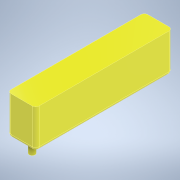
# Autodesk Inventor part: Schmierung
Saved by Autodesk Inventor 2022 (Build 260153000, 153)
## iProperties
Created: 2023-01-30
Part Number: Schmierung
Material: Wasser
Document SubType Name: Modeling
Designer: Matias Nicky
Density: 0.9983 g/cm^3
Appearance: Gelb
Author: Matias Nicky
Autodesk Inventor part; units mm, degrees
ref_plane "YZ Plane" through (0, 0, 0) normal (1, 0, 0) x (0, 1, 0)
ref_plane "XZ Plane" through (0, 0, 0) normal (0, 1, 0) x (-1, 0, 0)
ref_plane "XY Plane" through (0, 0, 0) normal (0, 0, 1) x (1, 0, 0)
sketch "Skizze1" plane through (0, 0, 0) normal (0, 1, 0) x (-1, 0, 0)
  line L0 (-15, -97) -> (15, -97)
  line L1 (20, -92) -> (20, 92)
  line L2 (15, 97) -> (-15, 97)
  line L3 (-20, 92) -> (-20, -92)
  line L4 (-20, -97) -> (20, 97) construction
  line L5 (20, -97) -> (-20, 97) construction
  arc A0 (20, 95) -> (18, 97) centre (18, 95) ccw
  arc A1 (20, 92) -> (15, 97) centre (15, 92) ccw
  arc A2 (-15, 97) -> (-20, 92) centre (-15, 92) ccw
  arc A3 (-20, -92) -> (-15, -97) centre (-15, -92) ccw
  arc A4 (15, -97) -> (20, -92) centre (15, -92) ccw
  point P0 (0, 0)
  dimension "d0" = 40
  dimension "d1" = 194
  dimension "d3" = 5
  dimension "d4" = 5
  constraints: 12 end point, 10 point on circle, 10 point on line, 10 tangent, 5 centre point, 2 equal radius, 2 midpoint, 2 parallel, 1 horizontal, 1 perpendicular
  measures "d0" distance of L5.end L4.end
  measures "d1" distance of L5.start L4.end
  measures "d3" radius of A1
  measures "d4" radius of A2
extrude "Extrusion1" add sketch "Skizze1" along normal blind 55
sketch "Skizze2" plane through (0, 0, 0) normal (0, -1, 0) x (1, 0, 0)
  circle A0 centre (0, 82) radius 4.188
  line L0 (-15, 97) -> (15, 97) projected
  point P0 (0, 0)
  dimension "d7" = 8.376
  dimension "d8" = 15
  constraints: 1 centre point
  measures "d7" diameter of A0
  measures "d8" distance from line of L0 A0.centre
extrude "Extrusion2" add sketch "Skizze2" along normal blind 18
fillet "Rundung1" radius 5 8 edges at (18.5355, 0, 95.5355) (20, 0, 0) (18.5355, 0, -95.5355) (0, 0, -97) (-18.5355, 0, -95.5355) (-20, 0, 0) (-18.5355, 0, 95.5355) (0, 0, 97)
